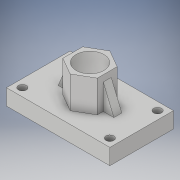
# Autodesk Inventor part: Задача 4
Saved by Autodesk Inventor 2019.1 (Build 231200000, 200)
## iProperties
Created: 2019-10-29
Part Number: Задача 4
Material: Типовые
Document SubType Name: Modeling
Designer: Stas
Density: 1 g/cm^3
Appearance: По умолчанию
Author: Stas
Autodesk Inventor part; units mm, degrees
ref_plane "YZ Plane" through (0, 0, 0) normal (1, 0, 0) x (0, 1, 0)
ref_plane "XZ Plane" through (0, 0, 0) normal (0, 1, 0) x (-1, 0, 0)
ref_plane "XY Plane" through (0, 0, 0) normal (0, 0, 1) x (1, 0, 0)
sketch "Эскиз1" plane through (0, 0, 0) normal (0, 1, 0) x (-1, 0, 0)
  line L0 (-65, -40) -> (65, -40)
  line L1 (65, -40) -> (65, 40)
  line L2 (65, 40) -> (-65, 40)
  line L3 (-65, 40) -> (-65, -40)
  circle A0 centre (55, -30) radius 5
  circle A1 centre (-55, -30) radius 5
  circle A2 centre (55, 30) radius 5
  circle A3 centre (-55, 30) radius 5
  point P0 (0, 0)
  constraints: 8 end point, 4 centre point, 2 parallel, 1 horizontal, 1 perpendicular
extrude "Выдавливание1" add sketch "Эскиз1" along normal blind 20
sketch "Эскиз2" plane through (0, 20, 0) normal (0, 1, 0) x (1, 0, 0)
  line L0 (0, -25) -> (-21.6506, -12.5)
  line L1 (-21.6506, -12.5) -> (-21.6506, 12.5)
  line L2 (-21.6506, 12.5) -> (0, 25)
  line L3 (0, 25) -> (21.6506, 12.5)
  line L4 (21.6506, 12.5) -> (21.6506, -12.5)
  line L5 (21.6506, -12.5) -> (0, -25)
  point P0 (0, 0)
  point P1 (0, 0)
  constraints: 12 end point, 1 coincident, 13 other
extrude "Выдавливание2" add sketch "Эскиз2" along normal blind 40
sketch "Эскиз3" plane through (0, 60, 0) normal (0, 1, 0) x (1, 0, 0)
  circle A0 centre (0, 0) radius 17.5
  constraints: 1 centre point
extrude "Выдавливание3" cut sketch "Эскиз3" against normal blind 30
sketch "Эскиз4" plane through (0, 30, 0) normal (0, 1, 0) x (1, 0, 0)
  circle A0 centre (0, 0) radius 17.5 projected
  line L0 (-10, 14.3614) -> (-10, -14.3614)
  line L1 (10, 0) -> (10, 14.3614)
  line L2 (10, 14.3614) -> (10, -14.3614)
  constraints: 6 end point, 4 point on circle, 1 point on line
extrude "Выдавливание4" cut sketch "Эскиз4" against normal blind 30 contours L1 L2 A0 L0
sketch "Эскиз5" plane through (0, 0, 0) normal (0, 0, 1) x (1, 0, 0)
  line L0 (10, 0) -> (-10, 0) projected
  line L1 (21.6506, 52) -> (35, 20)
  line L2 (-21.6506, 52) -> (-35, 20)
  point P0 (0, 0)
  point P1 (-21.6506, 20)
  point P2 (21.6506, 20)
  constraints: 4 end point
extrude "Ребро жесткости1" add sketch "Эскиз5" along normal mid plane 10 rib yes fills toward (-28.2792, 35.9807) open curves L2
mirror "Зеркальное отражение1" about plane through (0, 0, 0) normal (1, 0, 0) of "Ребро жесткости1"
